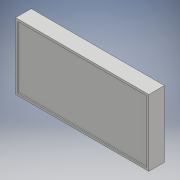
# Autodesk Inventor part: Base
Saved by Autodesk Inventor 2017 (Build 210142000, 142)
## iProperties
Created: 2016-11-26
Part Number: Base
Material: Generic
Document SubType Name: Modeling
Designer: umr
Density: 1 g/cm^3
Appearance: Default
Author: umr
Autodesk Inventor part; units mm, degrees
ref_plane "YZ Plane" through (0, 0, 0) normal (1, 0, 0) x (0, 1, 0)
ref_plane "XZ Plane" through (0, 0, 0) normal (0, 1, 0) x (-1, 0, 0)
ref_plane "XY Plane" through (0, 0, 0) normal (0, 0, 1) x (1, 0, 0)
sketch "Sketch1" plane through (0, 0, 0) normal (0, 1, 0) x (-1, 0, 0)
  line L0 (0, 0) -> (3000, 0)
  line L1 (3000, 0) -> (3000, -1500)
  line L2 (3000, -1500) -> (0, -1500)
  line L3 (0, -1500) -> (0, 0)
  dimension "d0" = 3000
  dimension "d1" = 1500
  constraints: 8 end point, 2 parallel, 1 horizontal, 1 perpendicular
  measures "d0" distance of L1.end L2.end
  measures "d1" distance of L0.end L1.end
extrude "Extrusion1" add sketch "Sketch1" along normal blind 350
sketch "Sketch2" plane through (0, 0, 0) normal (0, -1, 0) x (1, 0, 0)
  line L0 (-50, -50) -> (-2950, -50)
  line L1 (-2950, -50) -> (-2950, -1450)
  line L2 (-2950, -1450) -> (-50, -1450)
  line L3 (-50, -1450) -> (-50, -50)
  line L4 (0, 0) -> (-3000, 0) projected
  line L5 (0, -1500) -> (0, 0) projected
  dimension "d4" = 2900
  dimension "d5" = 1400
  dimension "d8" = 50
  dimension "d9" = 50
  constraints: 8 end point, 2 parallel, 1 horizontal, 1 perpendicular
  measures "d4" distance of L2.end L1.end
  measures "d5" distance of L1.end L0.end
  measures "d8" distance between parallel lines of L0 L4
  measures "d9" distance between parallel lines of L5 L3
extrude "Extrusion2" cut sketch "Sketch2" against normal blind 20
equation "\"d9\" = d8"
body "Solid1"
